Autodesk Fusion 360 part; units mm, degrees
(part 4 of 7)
  spline S47 degree 5 poles (-31.3994, -15.09) (-31.3967, -15.097) (-31.3914, -15.1111) (-31.3834, -15.1322) (-31.3727, -15.1603) (-31.3591, -15.1953) (-31.3454, -15.2302) (-31.3315, -15.265) (-31.3175, -15.2997) (-31.3034, -15.3343) (-31.2892, -15.3688) (-31.2748, -15.4031) (-31.2603, -15.4374) (-31.2457, -15.4715) (-31.2309, -15.5056) (-31.216, -15.5395) (-31.2009, -15.5733) (-31.1857, -15.607) (-31.1704, -15.6406) (-31.155, -15.674) (-31.1394, -15.7073) (-31.1236, -15.7406) (-31.1078, -15.7737) (-31.0917, -15.8066) (-31.0756, -15.8395) (-31.0593, -15.8722) (-31.0429, -15.9048) (-31.0263, -15.9373) (-31.0096, -15.9696) (-30.9927, -16.0018) (-30.9757, -16.0339) (-30.9586, -16.0658) (-30.9413, -16.0976) (-30.9238, -16.1293) (-30.9063, -16.1608) (-30.8885, -16.1922) (-30.8706, -16.2234) (-30.8526, -16.2545) (-30.8344, -16.2855) (-30.8161, -16.3163) (-30.7976, -16.3469) (-30.7789, -16.3774) (-30.7601, -16.4077) (-30.7411, -16.4379) (-30.722, -16.4679) (-30.7027, -16.4977) (-30.6833, -16.5274) (-30.6637, -16.5569) (-30.6439, -16.5863) (-30.6239, -16.6154) (-30.6038, -16.6444) (-30.5835, -16.6732) (-30.563, -16.7018) (-30.5423, -16.7301) (-30.5214, -16.7583) (-30.5003, -16.7862) (-30.4791, -16.814) (-30.4577, -16.8416) (-30.4361, -16.869) (-30.4144, -16.8962) (-30.3923, -16.9231) (-30.37, -16.9497) (-30.3474, -16.9759) (-30.3245, -17.0018) (-30.3014, -17.0274) (-30.2781, -17.0528) (-30.2546, -17.078) (-30.231, -17.103) (-30.2072, -17.1278) (-30.183, -17.1521) (-30.1582, -17.1757) (-30.1377, -17.1938) (-30.1219, -17.2068) (-30.1111, -17.2152) (-30.1057, -17.2194) knots -1 -1 -1 -1 -1 -1 -0.98571429 -0.97142857 -0.95714286 -0.94285714 -0.92857143 -0.91428571 -0.9 -0.88571429 -0.87142857 -0.85714286 -0.84285714 -0.82857143 -0.81428571 -0.8 -0.78571429 -0.77142857 -0.75714286 -0.74285714 -0.72857143 -0.71428571 -0.7 -0.68571429 -0.67142857 -0.65714286 -0.64285714 -0.62857143 -0.61428571 -0.6 -0.58571429 -0.57142857 -0.55714286 -0.54285714 -0.52857143 -0.51428571 -0.5 -0.48571429 -0.47142857 -0.45714286 -0.44285714 -0.42857143 -0.41428571 -0.4 -0.38571429 -0.37142857 -0.35714286 -0.34285714 -0.32857143 -0.31428571 -0.3 -0.28571429 -0.27142857 -0.25714286 -0.24285714 -0.22857143 -0.21428571 -0.2 -0.18571429 -0.17142857 -0.15714286 -0.14285714 -0.12857143 -0.11428571 -0.1 -0.08571429 -0.07142857 -0.05714286 -0.04285714 -0.02857143 -0.01428571 0 0 0 0 0 0
  line L47 (-30.1057, -17.2194) -> (-30.0219, -17.2834)
  arc A95 (-29.9186, -17.9712) -> (-30.0219, -17.2834) centre (-30.3255, -17.6807) ccw
  arc A96 (-29.9186, -17.9712) -> (-30.1974, -18.3752) centre (-17.3506, -26.9445) ccw
  arc A97 (-30.8771, -18.5225) -> (-30.1974, -18.3752) centre (-30.6134, -18.0977) ccw
  line L48 (-30.8771, -18.5225) -> (-30.9667, -18.4669)
  spline S48 degree 5 poles (-30.9667, -18.4669) (-30.9726, -18.4632) (-30.9843, -18.4562) (-31.002, -18.446) (-31.0262, -18.4333) (-31.0571, -18.4184) (-31.0884, -18.4045) (-31.12, -18.391) (-31.1518, -18.3778) (-31.1837, -18.3648) (-31.2157, -18.3519) (-31.2478, -18.3394) (-31.2802, -18.3272) (-31.3127, -18.3153) (-31.3455, -18.3039) (-31.3784, -18.2928) (-31.4115, -18.2821) (-31.4448, -18.2717) (-31.4782, -18.2614) (-31.5117, -18.2514) (-31.5453, -18.2417) (-31.5791, -18.2321) (-31.6129, -18.2228) (-31.6469, -18.2138) (-31.681, -18.205) (-31.7152, -18.1965) (-31.7496, -18.1882) (-31.784, -18.1801) (-31.8186, -18.1722) (-31.8532, -18.1645) (-31.888, -18.1571) (-31.9228, -18.1498) (-31.9577, -18.1428) (-31.9928, -18.1359) (-32.0279, -18.1293) (-32.0631, -18.1229) (-32.0984, -18.1167) (-32.1338, -18.1106) (-32.1692, -18.1048) (-32.2048, -18.0991) (-32.2404, -18.0937) (-32.2761, -18.0884) (-32.3119, -18.0833) (-32.3478, -18.0785) (-32.3837, -18.0737) (-32.4198, -18.0692) (-32.4558, -18.0649) (-32.492, -18.0607) (-32.5282, -18.0567) (-32.5646, -18.0529) (-32.6009, -18.0493) (-32.6374, -18.0459) (-32.6739, -18.0426) (-32.7104, -18.0395) (-32.7471, -18.0365) (-32.7838, -18.0338) (-32.8206, -18.0312) (-32.8574, -18.0288) (-32.8943, -18.0265) (-32.9312, -18.0244) (-32.9682, -18.0225) (-33.0053, -18.0208) (-33.0424, -18.0192) (-33.0796, -18.0178) (-33.1168, -18.0165) (-33.1541, -18.0154) (-33.1914, -18.0145) (-33.2288, -18.0137) (-33.2663, -18.0131) (-33.3038, -18.0127) (-33.3413, -18.0124) (-33.3714, -18.0123) (-33.394, -18.0123) (-33.409, -18.0123) (-33.4166, -18.0123) knots 0 0 0 0 0 0 0.01428571 0.02857143 0.04285714 0.05714286 0.07142857 0.08571429 0.1 0.11428571 0.12857143 0.14285714 0.15714286 0.17142857 0.18571429 0.2 0.21428571 0.22857143 0.24285714 0.25714286 0.27142857 0.28571429 0.3 0.31428571 0.32857143 0.34285714 0.35714286 0.37142857 0.38571429 0.4 0.41428571 0.42857143 0.44285714 0.45714286 0.47142857 0.48571429 0.5 0.51428571 0.52857143 0.54285714 0.55714286 0.57142857 0.58571429 0.6 0.61428571 0.62857143 0.64285714 0.65714286 0.67142857 0.68571429 0.7 0.71428571 0.72857143 0.74285714 0.75714286 0.77142857 0.78571429 0.8 0.81428571 0.82857143 0.84285714 0.85714286 0.87142857 0.88571429 0.9 0.91428571 0.92857143 0.94285714 0.95714286 0.97142857 0.98571429 1 1 1 1 1 1
  arc A98 (-33.4166, -18.0123) -> (-33.8281, -18.7965) centre (-17.3506, -26.9445) ccw
  spline S49 degree 5 poles (-33.8281, -18.7965) (-33.8239, -18.8027) (-33.8153, -18.8152) (-33.8025, -18.8337) (-33.7853, -18.8584) (-33.7638, -18.8892) (-33.7421, -18.9198) (-33.7203, -18.9502) (-33.6985, -18.9806) (-33.6765, -19.0108) (-33.6544, -19.0408) (-33.6322, -19.0708) (-33.6099, -19.1006) (-33.5876, -19.1302) (-33.5651, -19.1597) (-33.5425, -19.1891) (-33.5198, -19.2183) (-33.497, -19.2474) (-33.474, -19.2763) (-33.451, -19.3051) (-33.4279, -19.3337) (-33.4047, -19.3622) (-33.3814, -19.3906) (-33.3579, -19.4187) (-33.3344, -19.4468) (-33.3107, -19.4746) (-33.287, -19.5024) (-33.2631, -19.5299) (-33.2391, -19.5573) (-33.2151, -19.5846) (-33.1909, -19.6116) (-33.1666, -19.6385) (-33.1422, -19.6653) (-33.1177, -19.6918) (-33.0931, -19.7182) (-33.0683, -19.7445) (-33.0435, -19.7705) (-33.0185, -19.7964) (-32.9935, -19.8221) (-32.9683, -19.8476) (-32.943, -19.8729) (-32.9176, -19.8981) (-32.8921, -19.923) (-32.8664, -19.9478) (-32.8407, -19.9723) (-32.8148, -19.9967) (-32.7888, -20.0208) (-32.7627, -20.0448) (-32.7365, -20.0685) (-32.7101, -20.0921) (-32.6837, -20.1154) (-32.657, -20.1385) (-32.6303, -20.1613) (-32.6034, -20.1839) (-32.5764, -20.2062) (-32.5493, -20.2284) (-32.522, -20.2503) (-32.4946, -20.2719) (-32.4671, -20.2934) (-32.4395, -20.3145) (-32.4117, -20.3354) (-32.3836, -20.3558) (-32.3554, -20.3759) (-32.327, -20.3956) (-32.2984, -20.4149) (-32.2697, -20.434) (-32.2408, -20.4528) (-32.2119, -20.4715) (-32.1829, -20.4898) (-32.1536, -20.5076) (-32.1239, -20.5246) (-32.0996, -20.5373) (-32.0812, -20.5461) (-32.0687, -20.5517) (-32.0624, -20.5545) knots -1 -1 -1 -1 -1 -1 -0.98571429 -0.97142857 -0.95714286 -0.94285714 -0.92857143 -0.91428571 -0.9 -0.88571429 -0.87142857 -0.85714286 -0.84285714 -0.82857143 -0.81428571 -0.8 -0.78571429 -0.77142857 -0.75714286 -0.74285714 -0.72857143 -0.71428571 -0.7 -0.68571429 -0.67142857 -0.65714286 -0.64285714 -0.62857143 -0.61428571 -0.6 -0.58571429 -0.57142857 -0.55714286 -0.54285714 -0.52857143 -0.51428571 -0.5 -0.48571429 -0.47142857 -0.45714286 -0.44285714 -0.42857143 -0.41428571 -0.4 -0.38571429 -0.37142857 -0.35714286 -0.34285714 -0.32857143 -0.31428571 -0.3 -0.28571429 -0.27142857 -0.25714286 -0.24285714 -0.22857143 -0.21428571 -0.2 -0.18571429 -0.17142857 -0.15714286 -0.14285714 -0.12857143 -0.11428571 -0.1 -0.08571429 -0.07142857 -0.05714286 -0.04285714 -0.02857143 -0.01428571 0 0 0 0 0 0
  line L49 (-32.0624, -20.5545) -> (-31.9657, -20.5966)
  arc A99 (-31.7009, -21.2397) -> (-31.9657, -20.5966) centre (-32.1655, -21.055) ccw
  arc A100 (-31.7009, -21.2397) -> (-31.8749, -21.6986) centre (-17.3506, -26.9445) ccw
  arc A101 (-32.4996, -22.0043) -> (-31.8749, -21.6986) centre (-32.3452, -21.5288) ccw
  line L50 (-32.4996, -22.0043) -> (-32.5999, -21.9718)
  spline S50 degree 5 poles (-32.5999, -21.9718) (-32.6064, -21.9696) (-32.6195, -21.9656) (-32.6392, -21.9599) (-32.6657, -21.9534) (-32.6992, -21.9464) (-32.733, -21.9403) (-32.7669, -21.9347) (-32.8009, -21.9295) (-32.835, -21.9245) (-32.8691, -21.9198) (-32.9033, -21.9153) (-32.9376, -21.9111) (-32.9721, -21.9074) (-33.0066, -21.9042) (-33.0413, -21.9013) (-33.076, -21.8988) (-33.1108, -21.8966) (-33.1457, -21.8947) (-33.1806, -21.893) (-33.2156, -21.8916) (-33.2506, -21.8904) (-33.2857, -21.8895) (-33.3209, -21.8888) (-33.3561, -21.8884) (-33.3914, -21.8883) (-33.4267, -21.8885) (-33.4621, -21.8889) (-33.4975, -21.8895) (-33.533, -21.8904) (-33.5685, -21.8914) (-33.6041, -21.8927) (-33.6397, -21.8942) (-33.6753, -21.896) (-33.711, -21.898) (-33.7467, -21.9001) (-33.7825, -21.9026) (-33.8183, -21.9052) (-33.8541, -21.908) (-33.89, -21.911) (-33.9259, -21.9142) (-33.9618, -21.9177) (-33.9978, -21.9213) (-34.0338, -21.9251) (-34.0698, -21.9292) (-34.1059, -21.9334) (-34.1419, -21.9378) (-34.1781, -21.9424) (-34.2142, -21.9472) (-34.2504, -21.9522) (-34.2865, -21.9574) (-34.3227, -21.9628) (-34.359, -21.9683) (-34.3952, -21.9741) (-34.4315, -21.98) (-34.4678, -21.9861) (-34.5041, -21.9924) (-34.5404, -21.9989) (-34.5768, -22.0055) (-34.6132, -22.0123) (-34.6496, -22.0193) (-34.686, -22.0265) (-34.7224, -22.0338) (-34.7588, -22.0413) (-34.7953, -22.049) (-34.8317, -22.0569) (-34.8682, -22.0649) (-34.9047, -22.0731) (-34.9412, -22.0815) (-34.9777, -22.09) (-35.0142, -22.0988) (-35.0435, -22.1058) (-35.0654, -22.1112) (-35.08, -22.1149) (-35.0873, -22.1167) knots 0 0 0 0 0 0 0.01428571 0.02857143 0.04285714 0.05714286 0.07142857 0.08571429 0.1 0.11428571 0.12857143 0.14285714 0.15714286 0.17142857 0.18571429 0.2 0.21428571 0.22857143 0.24285714 0.25714286 0.27142857 0.28571429 0.3 0.31428571 0.32857143 0.34285714 0.35714286 0.37142857 0.38571429 0.4 0.41428571 0.42857143 0.44285714 0.45714286 0.47142857 0.48571429 0.5 0.51428571 0.52857143 0.54285714 0.55714286 0.57142857 0.58571429 0.6 0.61428571 0.62857143 0.64285714 0.65714286 0.67142857 0.68571429 0.7 0.71428571 0.72857143 0.74285714 0.75714286 0.77142857 0.78571429 0.8 0.81428571 0.82857143 0.84285714 0.85714286 0.87142857 0.88571429 0.9 0.91428571 0.92857143 0.94285714 0.95714286 0.97142857 0.98571429 1 1 1 1 1 1
  arc A102 (-35.0873, -22.1167) -> (-35.2993, -22.9766) centre (-17.3506, -26.9445) ccw
  spline S51 degree 5 poles (-35.2993, -22.9766) (-35.2936, -22.9816) (-35.2824, -22.9916) (-35.2655, -23.0066) (-35.2429, -23.0265) (-35.2146, -23.0512) (-35.1862, -23.0757) (-35.1578, -23.1001) (-35.1293, -23.1243) (-35.1008, -23.1484) (-35.0721, -23.1723) (-35.0434, -23.196) (-35.0147, -23.2196) (-34.9858, -23.243) (-34.9569, -23.2663) (-34.9279, -23.2894) (-34.8989, -23.3123) (-34.8698, -23.3351) (-34.8406, -23.3577) (-34.8114, -23.3802) (-34.7821, -23.4024) (-34.7527, -23.4245) (-34.7233, -23.4465) (-34.6938, -23.4682) (-34.6642, -23.4898) (-34.6346, -23.5112) (-34.6049, -23.5324) (-34.5751, -23.5535) (-34.5453, -23.5744) (-34.5154, -23.595) (-34.4855, -23.6155) (-34.4554, -23.6358) (-34.4253, -23.656) (-34.3952, -23.6759) (-34.365, -23.6956) (-34.3347, -23.7152) (-34.3043, -23.7345) (-34.2739, -23.7537) (-34.2434, -23.7726) (-34.2129, -23.7914) (-34.1822, -23.8099) (-34.1516, -23.8283) (-34.1208, -23.8464) (-34.09, -23.8643) (-34.0591, -23.8819) (-34.0282, -23.8994) (-33.9971, -23.9166) (-33.9661, -23.9336) (-33.9349, -23.9504) (-33.9037, -23.967) (-33.8724, -23.9833) (-33.8411, -23.9993) (-33.8096, -24.0151) (-33.7781, -24.0306) (-33.7465, -24.0458) (-33.7149, -24.0608) (-33.6832, -24.0755) (-33.6514, -24.09) (-33.6196, -24.1043) (-33.5877, -24.1182) (-33.5557, -24.1318) (-33.5236, -24.1449) (-33.4914, -24.1577) (-33.4591, -24.17) (-33.4267, -24.1819) (-33.3942, -24.1935) (-33.3617, -24.2049) (-33.3292, -24.2161) (-33.2966, -24.227) (-33.2639, -24.2373) (-33.231, -24.2466) (-33.2044, -24.2531) (-33.1843, -24.2573) (-33.1709, -24.2598) (-33.1641, -24.2609) knots -1 -1 -1 -1 -1 -1 -0.98571429 -0.97142857 -0.95714286 -0.94285714 -0.92857143 -0.91428571 -0.9 -0.88571429 -0.87142857 -0.85714286 -0.84285714 -0.82857143 -0.81428571 -0.8 -0.78571429 -0.77142857 -0.75714286 -0.74285714 -0.72857143 -0.71428571 -0.7 -0.68571429 -0.67142857 -0.65714286 -0.64285714 -0.62857143 -0.61428571 -0.6 -0.58571429 -0.57142857 -0.55714286 -0.54285714 -0.52857143 -0.51428571 -0.5 -0.48571429 -0.47142857 -0.45714286 -0.44285714 -0.42857143 -0.41428571 -0.4 -0.38571429 -0.37142857 -0.35714286 -0.34285714 -0.32857143 -0.31428571 -0.3 -0.28571429 -0.27142857 -0.25714286 -0.24285714 -0.22857143 -0.21428571 -0.2 -0.18571429 -0.17142857 -0.15714286 -0.14285714 -0.12857143 -0.11428571 -0.1 -0.08571429 -0.07142857 -0.05714286 -0.04285714 -0.02857143 -0.01428571 0 0 0 0 0 0
  line L51 (-33.1641, -24.2609) -> (-33.0602, -24.2787)
  arc A103 (-32.6491, -24.8397) -> (-33.0602, -24.2787) centre (-33.1444, -24.7715) ccw
  circle A104 centre (-17.3506, -26.9445) radius 2.7
  circle A105 centre (-17.3506, -26.9445) radius 2.7
  circle A106 centre (-17.3506, -26.9445) radius 2.7
  circle A107 centre (-17.3506, -26.9445) radius 4.25
  dimension "d37" = 8.5
  constraint concentric A0 A105
  constraint concentric A105 A106
  constraint concentric A105 A107
  measures "d37" diameter of A107
sketch "Sketch2 (2)" plane through (0, 0, 0) normal (0, 1, 0) x (1, 0, 0)
  circle A0 centre (-38.9137, -5.4395) radius 4.5
  circle A1 centre (-38.9137, -5.4395) radius 6.5
  dimension "d52" = 9
  dimension "d53" = 13
  constraint concentric A0 A1
  measures "d52" diameter of A0
  measures "d53" diameter of A1
extrude "Extrude1'" add sketch "Sketch2 (2)" along normal blind 107 separate body makes body 2
move_body "Move1" bodies 2 to x (0.996195, 0, -0.087156) y (0, 1, 0) z (0.087156, 0, 0.996195) at (25.7661, 0, -8.7245)
move_body "Move2" bodies 2 to x (1, 0, 0) y (0, 1, 0) z (0, 0, 1) at (0, -2, 0)
combine "Combine1" operation add target body 2 tool bodies 1
sketch "Sketch3" plane through (0, 0, 0) normal (1, 0, 0) x (0, 1, 0)
  line L0 (105.0534, -1.0193) -> (-2.1023, -1.0193)
  circle A0 centre (96.2618, -1.0193) radius 1.5
  circle A1 centre (83.5203, -1.0193) radius 1.375
  circle A2 centre (73.2634, -1.0193) radius 1.25
  circle A3 centre (64.1533, -1.0193) radius 1
  circle A4 centre (54.852, -1.0193) radius 1.5
  circle A5 centre (47.2708, -1.0193) radius 1.55
  circle A6 centre (39.3074, -1.0193) radius 1.375
  circle A7 centre (30.7706, -1.0193) radius 1.25
  circle A8 centre (22.0427, -1.0193) radius 1
  circle A9 centre (12.1681, -1.0193) radius 1.5
  circle A10 centre (4.0136, -1.0193) radius 1.5
  dimension "d56" = 3
  dimension "d57" = 2.75
  dimension "d58" = 2.5
  dimension "d59" = 2
  dimension "d60" = 3
  dimension "d61" = 3.1
  dimension "d62" = 2.75
  dimension "d63" = 2.5
  dimension "d64" = 2
  dimension "d65" = 3
  dimension "d66" = 3
  constraint horizontal L0
  constraint coincident L0 A0.centre
  constraint coincident L0 A1.centre
  constraint coincident L0 A2.centre
  constraint coincident L0 A3.centre
  constraint coincident L0 A4.centre
  constraint coincident L0 A5.centre
  constraint coincident L0 A6.centre
  constraint coincident L0 A7.centre
  constraint coincident L0 A8.centre
  constraint coincident L0 A9.centre
  constraint coincident L0 A10.centre
  measures "d56" diameter of A0
  measures "d57" diameter of A1
  measures "d58" diameter of A2
  measures "d59" diameter of A3
  measures "d60" diameter of A4
  measures "d61" diameter of A5
  measures "d62" diameter of A6
  measures "d63" diameter of A7
  measures "d64" diameter of A8
  measures "d65" diameter of A9
  measures "d66" diameter of A10
extrude "Extrude2" cut sketch "Sketch3" against normal blind 17 from surface at -10 bodies 2
component "Rack; Circular Pitch: 4.12283 mm; Num Teeth: 26; Pressure Angle: 20 deg; Backlash: 0.12 mm;" placed x (1, 0, 0) y (0, 1, 0) z (0, 0, 1) at (0, 0, 0)

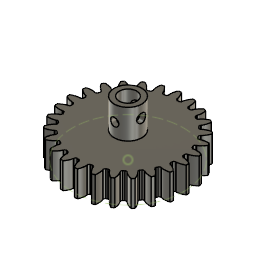
design "Pinion Gear (26t)"
description: Spur Gear; Module: 1.313; Num Teeth: 26; Pressure Angle: 20.0; Backlash: 0.12 mm
Autodesk Fusion 360 part; units mm, degrees
sketch "Sketch1" plane through (0, 0, 0) normal (0, 0, 1) x (1, 0, 0) in component "Spur Gear (26 teeth)"
  circle A0 centre (0, 0) radius 15.4426
  circle A1 centre (0, 0) radius 2.7
extrude "Extrude1" add sketch "Sketch1" along normal blind 8 in component "Spur Gear (26 teeth)"
sketch "Sketch2" plane through (0, 0, 0) normal (0, 0, 1) x (1, 0, 0) in component "Spur Gear (26 teeth)"
  spline S0 degree 5 poles (15.9962, -1.1788) (16.0031, -1.1793) (16.0167, -1.1802) (16.0372, -1.1809) (16.0645, -1.181) (16.0987, -1.1797) (16.1329, -1.1776) (16.1672, -1.1748) (16.2015, -1.1717) (16.2358, -1.1684) (16.27, -1.1649) (16.3044, -1.1611) (16.3387, -1.1569) (16.373, -1.1522) (16.4073, -1.1471) (16.4416, -1.1416) (16.4759, -1.1357) (16.5102, -1.1295) (16.5446, -1.123) (16.5789, -1.1163) (16.6132, -1.1094) (16.6475, -1.1021) (16.6818, -1.0946) (16.7161, -1.0868) (16.7504, -1.0788) (16.7846, -1.0704) (16.8189, -1.0618) (16.8532, -1.053) (16.8874, -1.0439) (16.9217, -1.0346) (16.9559, -1.025) (16.9901, -1.0153) (17.0243, -1.0053) (17.0585, -0.995) (17.0927, -0.9846) (17.1268, -0.9739) (17.161, -0.963) (17.1951, -0.9519) (17.2292, -0.9406) (17.2633, -0.9291) (17.2974, -0.9174) (17.3315, -0.9054) (17.3656, -0.8933) (17.3996, -0.8809) (17.4336, -0.8684) (17.4676, -0.8557) (17.5016, -0.8428) (17.5355, -0.8296) (17.5695, -0.8163) (17.6034, -0.8028) (17.6373, -0.7891) (17.6711, -0.7752) (17.705, -0.7612) (17.7388, -0.7469) (17.7726, -0.7325) (17.8064, -0.7179) (17.8402, -0.7031) (17.8739, -0.6881) (17.9076, -0.673) (17.9413, -0.6577) (17.9749, -0.6422) (18.0086, -0.6265) (18.0422, -0.6106) (18.0758, -0.5946) (18.1093, -0.5784) (18.1428, -0.5621) (18.1763, -0.5455) (18.2098, -0.5288) (18.2432, -0.512) (18.2766, -0.4949) (18.31, -0.4778) (18.3367, -0.4639) (18.3567, -0.4534) (18.37, -0.4463) (18.3767, -0.4428) knots 0 0 0 0 0 0 0.01428571 0.02857143 0.04285714 0.05714286 0.07142857 0.08571429 0.1 0.11428571 0.12857143 0.14285714 0.15714286 0.17142857 0.18571429 0.2 0.21428571 0.22857143 0.24285714 0.25714286 0.27142857 0.28571429 0.3 0.31428571 0.32857143 0.34285714 0.35714286 0.37142857 0.38571429 0.4 0.41428571 0.42857143 0.44285714 0.45714286 0.47142857 0.48571429 0.5 0.51428571 0.52857143 0.54285714 0.55714286 0.57142857 0.58571429 0.6 0.61428571 0.62857143 0.64285714 0.65714286 0.67142857 0.68571429 0.7 0.71428571 0.72857143 0.74285714 0.75714286 0.77142857 0.78571429 0.8 0.81428571 0.82857143 0.84285714 0.85714286 0.87142857 0.88571429 0.9 0.91428571 0.92857143 0.94285714 0.95714286 0.97142857 0.98571429 1 1 1 1 1 1
  spline S1 degree 5 poles (15.9962, 1.1788) (16.0031, 1.1793) (16.0167, 1.1802) (16.0372, 1.1809) (16.0645, 1.181) (16.0987, 1.1797) (16.1329, 1.1776) (16.1672, 1.1748) (16.2015, 1.1717) (16.2358, 1.1684) (16.27, 1.1649) (16.3044, 1.1611) (16.3387, 1.1569) (16.373, 1.1522) (16.4073, 1.1471) (16.4416, 1.1416) (16.4759, 1.1357) (16.5102, 1.1295) (16.5446, 1.123) (16.5789, 1.1163) (16.6132, 1.1094) (16.6475, 1.1021) (16.6818, 1.0946) (16.7161, 1.0868) (16.7504, 1.0788) (16.7846, 1.0704) (16.8189, 1.0618) (16.8532, 1.053) (16.8874, 1.0439) (16.9217, 1.0346) (16.9559, 1.025) (16.9901, 1.0153) (17.0243, 1.0053) (17.0585, 0.995) (17.0927, 0.9846) (17.1268, 0.9739) (17.161, 0.963) (17.1951, 0.9519) (17.2292, 0.9406) (17.2633, 0.9291) (17.2974, 0.9174) (17.3315, 0.9054) (17.3656, 0.8933) (17.3996, 0.8809) (17.4336, 0.8684) (17.4676, 0.8557) (17.5016, 0.8428) (17.5355, 0.8296) (17.5695, 0.8163) (17.6034, 0.8028) (17.6373, 0.7891) (17.6711, 0.7752) (17.705, 0.7612) (17.7388, 0.7469) (17.7726, 0.7325) (17.8064, 0.7179) (17.8402, 0.7031) (17.8739, 0.6881) (17.9076, 0.673) (17.9413, 0.6577) (17.9749, 0.6422) (18.0086, 0.6265) (18.0422, 0.6106) (18.0758, 0.5946) (18.1093, 0.5784) (18.1428, 0.5621) (18.1763, 0.5455) (18.2098, 0.5288) (18.2432, 0.512) (18.2766, 0.4949) (18.31, 0.4778) (18.3367, 0.4639) (18.3567, 0.4534) (18.37, 0.4463) (18.3767, 0.4428) knots 0 0 0 0 0 0 0.01428571 0.02857143 0.04285714 0.05714286 0.07142857 0.08571429 0.1 0.11428571 0.12857143 0.14285714 0.15714286 0.17142857 0.18571429 0.2 0.21428571 0.22857143 0.24285714 0.25714286 0.27142857 0.28571429 0.3 0.31428571 0.32857143 0.34285714 0.35714286 0.37142857 0.38571429 0.4 0.41428571 0.42857143 0.44285714 0.45714286 0.47142857 0.48571429 0.5 0.51428571 0.52857143 0.54285714 0.55714286 0.57142857 0.58571429 0.6 0.61428571 0.62857143 0.64285714 0.65714286 0.67142857 0.68571429 0.7 0.71428571 0.72857143 0.74285714 0.75714286 0.77142857 0.78571429 0.8 0.81428571 0.82857143 0.84285714 0.85714286 0.87142857 0.88571429 0.9 0.91428571 0.92857143 0.94285714 0.95714286 0.97142857 0.98571429 1 1 1 1 1 1
  arc A0 (18.3767, -0.4428) -> (18.3767, 0.4428) centre (0, 0) ccw
  line L0 (15.3909, -1.135) -> (15.9962, -1.1788)
  line L1 (15.3909, 1.135) -> (15.9962, 1.1788)
  line L2 (15.3909, -1.135) -> (15.3909, 1.135)
  point P0 (16.1643, -1.175)
  point P1 (16.3333, -1.1575)
  point P2 (16.5029, -1.1308)
  point P3 (16.6728, -1.0965)
  point P4 (16.8431, -1.0555)
  point P5 (17.0136, -1.0084)
  point P6 (17.1843, -0.9554)
  point P7 (17.355, -0.897)
  point P8 (17.5256, -0.8334)
  point P9 (17.6962, -0.7648)
  point P10 (17.8667, -0.6913)
  point P11 (18.037, -0.6131)
  point P12 (18.207, -0.5302)
  point P13 (16.1643, 1.175)
  point P14 (16.3333, 1.1575)
  point P15 (16.5029, 1.1308)
  point P16 (16.6728, 1.0965)
  point P17 (16.8431, 1.0555)
  point P18 (17.0136, 1.0084)
  point P19 (17.1843, 0.9554)
  point P20 (17.355, 0.897)
  point P21 (17.5256, 0.8334)
  point P22 (17.6962, 0.7648)
  point P23 (17.8667, 0.6913)
  point P24 (18.037, 0.6131)
  point P25 (18.207, 0.5302)
extrude "Extrude2" add sketch "Sketch2" along normal blind 8 in component "Spur Gear (26 teeth)"
fillet "Fillet1" radius 0.5 2 edges at (15.4008, -1.1357, 4) (15.4008, 1.1357, 4) in component "Spur Gear (26 teeth)"
pattern_circular "C-Pattern1" count 26 over 360 about axis through (0, 0, 0) along (0, 0, 1) of "Extrude2", "Fillet1" in component "Spur Gear (26 teeth)"
sketch "Sketch3" plane through (0, 0, 0) normal (0, 0, 1) x (1, 0, 0) in component "Spur Gear (26 teeth)"
  circle A0 centre (0, 0) radius 17.069 construction
sketch "Sketch1 (2)" plane through (0, 0, 8) normal (0, 0, 1) x (-1, 0, 0)
  arc A0 (-32.6491, -24.8397) -> (-32.7083, -25.327) centre (-17.3506, -26.9445) ccw
  arc A1 (-33.2417, -25.7733) -> (-32.7083, -25.327) centre (-33.2055, -25.2746) ccw
  line L0 (-33.2417, -25.7733) -> (-33.3469, -25.7656)
  spline S0 degree 5 poles (-33.3469, -25.7656) (-33.3537, -25.7652) (-33.3673, -25.7643) (-33.3878, -25.7636) (-33.4151, -25.7635) (-33.4493, -25.7648) (-33.4836, -25.7669) (-33.5178, -25.7697) (-33.5521, -25.7728) (-33.5864, -25.7761) (-33.6207, -25.7796) (-33.655, -25.7834) (-33.6893, -25.7876) (-33.7236, -25.7922) (-33.7579, -25.7974) (-33.7922, -25.8029) (-33.8265, -25.8088) (-33.8609, -25.815) (-33.8952, -25.8214) (-33.9295, -25.8282) (-33.9638, -25.8351) (-33.9981, -25.8424) (-34.0324, -25.8499) (-34.0667, -25.8577) (-34.101, -25.8657) (-34.1353, -25.8741) (-34.1695, -25.8827) (-34.2038, -25.8915) (-34.238, -25.9006) (-34.2723, -25.9099) (-34.3065, -25.9194) (-34.3407, -25.9292) (-34.3749, -25.9392) (-34.4091, -25.9494) (-34.4433, -25.9599) (-34.4775, -25.9706) (-34.5116, -25.9815) (-34.5457, -25.9926) (-34.5799, -26.0039) (-34.614, -26.0154) (-34.6481, -26.0271) (-34.6821, -26.0391) (-34.7162, -26.0512) (-34.7502, -26.0635) (-34.7842, -26.0761) (-34.8182, -26.0888) (-34.8522, -26.1017) (-34.8861, -26.1149) (-34.9201, -26.1282) (-34.954, -26.1417) (-34.9879, -26.1554) (-35.0218, -26.1692) (-35.0556, -26.1833) (-35.0894, -26.1976) (-35.1232, -26.212) (-35.157, -26.2266) (-35.1908, -26.2414) (-35.2245, -26.2564) (-35.2582, -26.2715) (-35.2919, -26.2868) (-35.3256, -26.3023) (-35.3592, -26.318) (-35.3928, -26.3339) (-35.4264, -26.3499) (-35.4599, -26.3661) (-35.4934, -26.3824) (-35.5269, -26.399) (-35.5604, -26.4157) (-35.5938, -26.4325) (-35.6272, -26.4495) (-35.6606, -26.4667) (-35.6873, -26.4806) (-35.7073, -26.4911) (-35.7206, -26.4981) (-35.7273, -26.5017) knots 0 0 0 0 0 0 0.01428571 0.02857143 0.04285714 0.05714286 0.07142857 0.08571429 0.1 0.11428571 0.12857143 0.14285714 0.15714286 0.17142857 0.18571429 0.2 0.21428571 0.22857143 0.24285714 0.25714286 0.27142857 0.28571429 0.3 0.31428571 0.32857143 0.34285714 0.35714286 0.37142857 0.38571429 0.4 0.41428571 0.42857143 0.44285714 0.45714286 0.47142857 0.48571429 0.5 0.51428571 0.52857143 0.54285714 0.55714286 0.57142857 0.58571429 0.6 0.61428571 0.62857143 0.64285714 0.65714286 0.67142857 0.68571429 0.7 0.71428571 0.72857143 0.74285714 0.75714286 0.77142857 0.78571429 0.8 0.81428571 0.82857143 0.84285714 0.85714286 0.87142857 0.88571429 0.9 0.91428571 0.92857143 0.94285714 0.95714286 0.97142857 0.98571429 1 1 1 1 1 1
  arc A2 (-35.7273, -26.5017) -> (-35.7273, -27.3873) centre (-17.3506, -26.9445) ccw
  spline S1 degree 5 poles (-35.7273, -27.3873) (-35.7206, -27.3908) (-35.7073, -27.3979) (-35.6873, -27.4084) (-35.6606, -27.4222) (-35.6272, -27.4394) (-35.5938, -27.4565) (-35.5604, -27.4733) (-35.5269, -27.49) (-35.4934, -27.5066) (-35.4599, -27.5229) (-35.4264, -27.5391) (-35.3928, -27.5551) (-35.3592, -27.571) (-35.3256, -27.5866) (-35.2919, -27.6021) (-35.2582, -27.6175) (-35.2245, -27.6326) (-35.1908, -27.6476) (-35.157, -27.6624) (-35.1232, -27.677) (-35.0894, -27.6914) (-35.0556, -27.7057) (-35.0218, -27.7197) (-34.9879, -27.7336) (-34.954, -27.7473) (-34.9201, -27.7608) (-34.8861, -27.7741) (-34.8522, -27.7872) (-34.8182, -27.8002) (-34.7842, -27.8129) (-34.7502, -27.8254) (-34.7162, -27.8378) (-34.6821, -27.8499) (-34.6481, -27.8618) (-34.614, -27.8736) (-34.5799, -27.8851) (-34.5457, -27.8964) (-34.5116, -27.9075) (-34.4775, -27.9184) (-34.4433, -27.9291) (-34.4091, -27.9395) (-34.3749, -27.9498) (-34.3407, -27.9598) (-34.3065, -27.9695) (-34.2723, -27.9791) (-34.238, -27.9884) (-34.2038, -27.9975) (-34.1695, -28.0063) (-34.1353, -28.0149) (-34.101, -28.0233) (-34.0667, -28.0313) (-34.0324, -28.0391) (-33.9981, -28.0466) (-33.9638, -28.0538) (-33.9295, -28.0608) (-33.8952, -28.0675) (-33.8609, -28.074) (-33.8265, -28.0802) (-33.7922, -28.0861) (-33.7579, -28.0916) (-33.7236, -28.0967) (-33.6893, -28.1014) (-33.655, -28.1056) (-33.6207, -28.1094) (-33.5864, -28.1129) (-33.5521, -28.1162) (-33.5178, -28.1193) (-33.4836, -28.1221) (-33.4493, -28.1242) (-33.4151, -28.1254) (-33.3878, -28.1254) (-33.3673, -28.1247) (-33.3537, -28.1238) (-33.3469, -28.1233) knots -1 -1 -1 -1 -1 -1 -0.98571429 -0.97142857 -0.95714286 -0.94285714 -0.92857143 -0.91428571 -0.9 -0.88571429 -0.87142857 -0.85714286 -0.84285714 -0.82857143 -0.81428571 -0.8 -0.78571429 -0.77142857 -0.75714286 -0.74285714 -0.72857143 -0.71428571 -0.7 -0.68571429 -0.67142857 -0.65714286 -0.64285714 -0.62857143 -0.61428571 -0.6 -0.58571429 -0.57142857 -0.55714286 -0.54285714 -0.52857143 -0.51428571 -0.5 -0.48571429 -0.47142857 -0.45714286 -0.44285714 -0.42857143 -0.41428571 -0.4 -0.38571429 -0.37142857 -0.35714286 -0.34285714 -0.32857143 -0.31428571 -0.3 -0.28571429 -0.27142857 -0.25714286 -0.24285714 -0.22857143 -0.21428571 -0.2 -0.18571429 -0.17142857 -0.15714286 -0.14285714 -0.12857143 -0.11428571 -0.1 -0.08571429 -0.07142857 -0.05714286 -0.04285714 -0.02857143 -0.01428571 0 0 0 0 0 0
  line L1 (-33.3469, -28.1233) -> (-33.2417, -28.1157)
  arc A3 (-32.7083, -28.562) -> (-33.2417, -28.1157) centre (-33.2055, -28.6144) ccw
  arc A4 (-32.7083, -28.562) -> (-32.6491, -29.0493) centre (-17.3506, -26.9445) ccw
  arc A5 (-33.0602, -29.6103) -> (-32.6491, -29.0493) centre (-33.1444, -29.1174) ccw
  line L2 (-33.0602, -29.6103) -> (-33.1641, -29.6281)
  spline S2 degree 5 poles (-33.1641, -29.6281) (-33.1709, -29.6292) (-33.1843, -29.6317) (-33.2044, -29.6358) (-33.231, -29.6423) (-33.2639, -29.6517) (-33.2966, -29.662) (-33.3292, -29.6729) (-33.3617, -29.6841) (-33.3942, -29.6955) (-33.4267, -29.7071) (-33.4591, -29.719) (-33.4914, -29.7313) (-33.5236, -29.744) (-33.5557, -29.7572) (-33.5877, -29.7708) (-33.6196, -29.7847) (-33.6514, -29.799) (-33.6832, -29.8135) (-33.7149, -29.8282) (-33.7465, -29.8432) (-33.7781, -29.8584) (-33.8096, -29.8739) (-33.8411, -29.8897) (-33.8724, -29.9057) (-33.9037, -29.922) (-33.9349, -29.9386) (-33.9661, -29.9553) (-33.9971, -29.9724) (-34.0282, -29.9896) (-34.0591, -30.007) (-34.09, -30.0247) (-34.1208, -30.0426) (-34.1516, -30.0607) (-34.1822, -30.0791) (-34.2129, -30.0976) (-34.2434, -30.1163) (-34.2739, -30.1353) (-34.3043, -30.1544) (-34.3347, -30.1738) (-34.365, -30.1933) (-34.3952, -30.2131) (-34.4253, -30.233) (-34.4554, -30.2531) (-34.4855, -30.2734) (-34.5154, -30.2939) (-34.5453, -30.3146) (-34.5751, -30.3355) (-34.6049, -30.3565) (-34.6346, -30.3778) (-34.6642, -30.3992) (-34.6938, -30.4208) (-34.7233, -30.4425) (-34.7527, -30.4644) (-34.7821, -30.4865) (-34.8114, -30.5088) (-34.8406, -30.5313) (-34.8698, -30.5539) (-34.8989, -30.5766) (-34.9279, -30.5996) (-34.9569, -30.6227) (-34.9858, -30.6459) (-35.0147, -30.6694) (-35.0434, -30.693) (-35.0721, -30.7167) (-35.1008, -30.7406) (-35.1293, -30.7647) (-35.1578, -30.7889) (-35.1862, -30.8133) (-35.2146, -30.8378) (-35.2429, -30.8625) (-35.2655, -30.8824) (-35.2824, -30.8973) (-35.2936, -30.9073) (-35.2993, -30.9124) knots 0 0 0 0 0 0 0.01428571 0.02857143 0.04285714 0.05714286 0.07142857 0.08571429 0.1 0.11428571 0.12857143 0.14285714 0.15714286 0.17142857 0.18571429 0.2 0.21428571 0.22857143 0.24285714 0.25714286 0.27142857 0.28571429 0.3 0.31428571 0.32857143 0.34285714 0.35714286 0.37142857 0.38571429 0.4 0.41428571 0.42857143 0.44285714 0.45714286 0.47142857 0.48571429 0.5 0.51428571 0.52857143 0.54285714 0.55714286 0.57142857 0.58571429 0.6 0.61428571 0.62857143 0.64285714 0.65714286 0.67142857 0.68571429 0.7 0.71428571 0.72857143 0.74285714 0.75714286 0.77142857 0.78571429 0.8 0.81428571 0.82857143 0.84285714 0.85714286 0.87142857 0.88571429 0.9 0.91428571 0.92857143 0.94285714 0.95714286 0.97142857 0.98571429 1 1 1 1 1 1
  arc A6 (-35.2993, -30.9124) -> (-35.0873, -31.7723) centre (-17.3506, -26.9445) ccw
  spline S3 degree 5 poles (-35.0873, -31.7723) (-35.08, -31.7741) (-35.0654, -31.7777) (-35.0435, -31.7831) (-35.0142, -31.7902) (-34.9777, -31.7989) (-34.9412, -31.8075) (-34.9047, -31.8158) (-34.8682, -31.824) (-34.8317, -31.8321) (-34.7953, -31.8399) (-34.7588, -31.8476) (-34.7224, -31.8552) (-34.686, -31.8625) (-34.6496, -31.8697) (-34.6132, -31.8767) (-34.5768, -31.8835) (-34.5404, -31.8901) (-34.5041, -31.8966) (-34.4678, -31.9029) (-34.4315, -31.909) (-34.3952, -31.9149) (-34.359, -31.9206) (-34.3227, -31.9262) (-34.2865, -31.9316) (-34.2504, -31.9367) (-34.2142, -31.9417) (-34.1781, -31.9465) (-34.1419, -31.9512) (-34.1059, -31.9556) (-34.0698, -31.9598) (-34.0338, -31.9638) (-33.9978, -31.9677) (-33.9618, -31.9713) (-33.9259, -31.9747) (-33.89, -31.978) (-33.8541, -31.981) (-33.8183, -31.9838) (-33.7825, -31.9864) (-33.7467, -31.9888) (-33.711, -31.991) (-33.6753, -31.993) (-33.6397, -31.9947) (-33.6041, -31.9963) (-33.5685, -31.9976) (-33.533, -31.9986) (-33.4975, -31.9995) (-33.4621, -32.0001) (-33.4267, -32.0005) (-33.3914, -32.0006) (-33.3561, -32.0005) (-33.3209, -32.0002) (-33.2857, -31.9995) (-33.2506, -31.9986) (-33.2156, -31.9974) (-33.1806, -31.996) (-33.1457, -31.9943) (-33.1108, -31.9923) (-33.076, -31.9902) (-33.0413, -31.9877) (-33.0066, -31.9848) (-32.9721, -31.9816) (-32.9376, -31.9779) (-32.9033, -31.9737) (-32.8691, -31.9692) (-32.835, -31.9644) (-32.8009, -31.9594) (-32.7669, -31.9542) (-32.733, -31.9487) (-32.6992, -31.9426) (-32.6657, -31.9356) (-32.6392, -31.929) (-32.6195, -31.9234) (-32.6064, -31.9193) (-32.5999, -31.9172) knots -1 -1 -1 -1 -1 -1 -0.98571429 -0.97142857 -0.95714286 -0.94285714 -0.92857143 -0.91428571 -0.9 -0.88571429 -0.87142857 -0.85714286 -0.84285714 -0.82857143 -0.81428571 -0.8 -0.78571429 -0.77142857 -0.75714286 -0.74285714 -0.72857143 -0.71428571 -0.7 -0.68571429 -0.67142857 -0.65714286 -0.64285714 -0.62857143 -0.61428571 -0.6 -0.58571429 -0.57142857 -0.55714286 -0.54285714 -0.52857143 -0.51428571 -0.5 -0.48571429 -0.47142857 -0.45714286 -0.44285714 -0.42857143 -0.41428571 -0.4 -0.38571429 -0.37142857 -0.35714286 -0.34285714 -0.32857143 -0.31428571 -0.3 -0.28571429 -0.27142857 -0.25714286 -0.24285714 -0.22857143 -0.21428571 -0.2 -0.18571429 -0.17142857 -0.15714286 -0.14285714 -0.12857143 -0.11428571 -0.1 -0.08571429 -0.07142857 -0.05714286 -0.04285714 -0.02857143 -0.01428571 0 0 0 0 0 0
  line L3 (-32.5999, -31.9172) -> (-32.4996, -31.8847)
  arc A7 (-31.8749, -32.1904) -> (-32.4996, -31.8847) centre (-32.3452, -32.3602) ccw
  arc A8 (-31.8749, -32.1904) -> (-31.7009, -32.6493) centre (-17.3506, -26.9445) ccw
  arc A9 (-31.9657, -33.2924) -> (-31.7009, -32.6493) centre (-32.1655, -32.834) ccw
  line L4 (-31.9657, -33.2924) -> (-32.0624, -33.3345)
  spline S4 degree 5 poles (-32.0624, -33.3345) (-32.0687, -33.3372) (-32.0812, -33.3428) (-32.0996, -33.3517) (-32.1239, -33.3644) (-32.1536, -33.3813) (-32.1829, -33.3992) (-32.2119, -33.4175) (-32.2408, -33.4362) (-32.2697, -33.455) (-32.2984, -33.4741) (-32.327, -33.4934) (-32.3554, -33.5131) (-32.3836, -33.5331) (-32.4117, -33.5536) (-32.4395, -33.5744) (-32.4671, -33.5956) (-32.4946, -33.617) (-32.522, -33.6387) (-32.5493, -33.6606) (-32.5764, -33.6827) (-32.6034, -33.7051) (-32.6303, -33.7277) (-32.657, -33.7505) (-32.6837, -33.7736) (-32.7101, -33.7969) (-32.7365, -33.8204) (-32.7627, -33.8442) (-32.7888, -33.8681) (-32.8148, -33.8923) (-32.8407, -33.9167) (-32.8664, -33.9412) (-32.8921, -33.966) (-32.9176, -33.9909) (-32.943, -34.016) (-32.9683, -34.0414) (-32.9935, -34.0669) (-33.0185, -34.0926) (-33.0435, -34.1185) (-33.0683, -34.1445) (-33.0931, -34.1707) (-33.1177, -34.1971) (-33.1422, -34.2237) (-33.1666, -34.2504) (-33.1909, -34.2773) (-33.2151, -34.3044) (-33.2391, -34.3317) (-33.2631, -34.3591) (-33.287, -34.3866) (-33.3107, -34.4143) (-33.3344, -34.4422) (-33.3579, -34.4702) (-33.3814, -34.4984) (-33.4047, -34.5268) (-33.4279, -34.5552) (-33.451, -34.5839) (-33.474, -34.6127) (-33.497, -34.6416) (-33.5198, -34.6707) (-33.5425, -34.6999) (-33.5651, -34.7293) (-33.5876, -34.7588) (-33.6099, -34.7884) (-33.6322, -34.8182) (-33.6544, -34.8481) (-33.6765, -34.8782) (-33.6985, -34.9084) (-33.7203, -34.9387) (-33.7421, -34.9692) (-33.7638, -34.9998) (-33.7853, -35.0305) (-33.8025, -35.0552) (-33.8153, -35.0738) (-33.8239, -35.0862) (-33.8281, -35.0924) knots 0 0 0 0 0 0 0.01428571 0.02857143 0.04285714 0.05714286 0.07142857 0.08571429 0.1 0.11428571 0.12857143 0.14285714 0.15714286 0.17142857 0.18571429 0.2 0.21428571 0.22857143 0.24285714 0.25714286 0.27142857 0.28571429 0.3 0.31428571 0.32857143 0.34285714 0.35714286 0.37142857 0.38571429 0.4 0.41428571 0.42857143 0.44285714 0.45714286 0.47142857 0.48571429 0.5 0.51428571 0.52857143 0.54285714 0.55714286 0.57142857 0.58571429 0.6 0.61428571 0.62857143 0.64285714 0.65714286 0.67142857 0.68571429 0.7 0.71428571 0.72857143 0.74285714 0.75714286 0.77142857 0.78571429 0.8 0.81428571 0.82857143 0.84285714 0.85714286 0.87142857 0.88571429 0.9 0.91428571 0.92857143 0.94285714 0.95714286 0.97142857 0.98571429 1 1 1 1 1 1
  arc A10 (-33.8281, -35.0924) -> (-33.4166, -35.8767) centre (-17.3506, -26.9445) ccw
  spline S5 degree 5 poles (-33.4166, -35.8767) (-33.409, -35.8767) (-33.394, -35.8767) (-33.3714, -35.8767) (-33.3413, -35.8766) (-33.3038, -35.8763) (-33.2663, -35.8759) (-33.2288, -35.8753) (-33.1914, -35.8745) (-33.1541, -35.8736) (-33.1168, -35.8725) (-33.0796, -35.8712) (-33.0424, -35.8698) (-33.0053, -35.8682) (-32.9682, -35.8665) (-32.9312, -35.8645) (-32.8943, -35.8625) (-32.8574, -35.8602) (-32.8206, -35.8578) (-32.7838, -35.8552) (-32.7471, -35.8524) (-32.7104, -35.8495) (-32.6739, -35.8464) (-32.6374, -35.8431) (-32.6009, -35.8397) (-32.5646, -35.836) (-32.5282, -35.8322) (-32.492, -35.8283) (-32.4558, -35.8241) (-32.4198, -35.8198) (-32.3837, -35.8152) (-32.3478, -35.8105) (-32.3119, -35.8056) (-32.2761, -35.8006) (-32.2404, -35.7953) (-32.2048, -35.7898) (-32.1692, -35.7842) (-32.1338, -35.7783) (-32.0984, -35.7723) (-32.0631, -35.7661) (-32.0279, -35.7597) (-31.9928, -35.753) (-31.9577, -35.7462) (-31.9228, -35.7392) (-31.888, -35.7319) (-31.8532, -35.7245) (-31.8186, -35.7168) (-31.784, -35.7089) (-31.7496, -35.7008) (-31.7152, -35.6925) (-31.681, -35.684) (-31.6469, -35.6752) (-31.6129, -35.6661) (-31.5791, -35.6568) (-31.5453, -35.6473) (-31.5117, -35.6375) (-31.4782, -35.6275) (-31.4448, -35.6173) (-31.4115, -35.6069) (-31.3784, -35.5961) (-31.3455, -35.5851) (-31.3127, -35.5736) (-31.2802, -35.5618) (-31.2478, -35.5496) (-31.2157, -35.537) (-31.1837, -35.5242) (-31.1518, -35.5112) (-31.12, -35.498) (-31.0884, -35.4845) (-31.0571, -35.4705) (-31.0262, -35.4557) (-31.002, -35.443) (-30.9843, -35.4328) (-30.9726, -35.4257) (-30.9667, -35.4221) knots -1 -1 -1 -1 -1 -1 -0.98571429 -0.97142857 -0.95714286 -0.94285714 -0.92857143 -0.91428571 -0.9 -0.88571429 -0.87142857 -0.85714286 -0.84285714 -0.82857143 -0.81428571 -0.8 -0.78571429 -0.77142857 -0.75714286 -0.74285714 -0.72857143 -0.71428571 -0.7 -0.68571429 -0.67142857 -0.65714286 -0.64285714 -0.62857143 -0.61428571 -0.6 -0.58571429 -0.57142857 -0.55714286 -0.54285714 -0.52857143 -0.51428571 -0.5 -0.48571429 -0.47142857 -0.45714286 -0.44285714 -0.42857143 -0.41428571 -0.4 -0.38571429 -0.37142857 -0.35714286 -0.34285714 -0.32857143 -0.31428571 -0.3 -0.28571429 -0.27142857 -0.25714286 -0.24285714 -0.22857143 -0.21428571 -0.2 -0.18571429 -0.17142857 -0.15714286 -0.14285714 -0.12857143 -0.11428571 -0.1 -0.08571429 -0.07142857 -0.05714286 -0.04285714 -0.02857143 -0.01428571 0 0 0 0 0 0
  line L5 (-30.9667, -35.4221) -> (-30.8771, -35.3665)
  arc A11 (-30.1974, -35.5138) -> (-30.8771, -35.3665) centre (-30.6134, -35.7913) ccw
  arc A12 (-30.1974, -35.5138) -> (-29.9186, -35.9178) centre (-17.3506, -26.9445) ccw
  arc A13 (-30.0219, -36.6055) -> (-29.9186, -35.9178) centre (-30.3255, -36.2083) ccw
  line L6 (-30.0219, -36.6055) -> (-30.1057, -36.6696)
  spline S6 degree 5 poles (-30.1057, -36.6696) (-30.1111, -36.6737) (-30.1219, -36.6822) (-30.1377, -36.6952) (-30.1582, -36.7133) (-30.183, -36.7369) (-30.2072, -36.7612) (-30.231, -36.786) (-30.2546, -36.811) (-30.2781, -36.8362) (-30.3014, -36.8616) (-30.3245, -36.8872) (-30.3474, -36.9131) (-30.37, -36.9393) (-30.3923, -36.9659) (-30.4144, -36.9928) (-30.4361, -37.02) (-30.4577, -37.0474) (-30.4791, -37.075) (-30.5003, -37.1027) (-30.5214, -37.1307) (-30.5423, -37.1589) (-30.563, -37.1872) (-30.5835, -37.2158) (-30.6038, -37.2446) (-30.6239, -37.2735) (-30.6439, -37.3027) (-30.6637, -37.332) (-30.6833, -37.3616) (-30.7027, -37.3912) (-30.722, -37.4211) (-30.7411, -37.4511) (-30.7601, -37.4812) (-30.7789, -37.5116) (-30.7976, -37.5421) (-30.8161, -37.5727) (-30.8344, -37.6035) (-30.8526, -37.6344) (-30.8706, -37.6655) (-30.8885, -37.6968) (-30.9063, -37.7282) (-30.9238, -37.7597) (-30.9413, -37.7913) (-30.9586, -37.8232) (-30.9757, -37.8551) (-30.9927, -37.8872) (-31.0096, -37.9194) (-31.0263, -37.9517) (-31.0429, -37.9842) (-31.0593, -38.0168) (-31.0756, -38.0495) (-31.0917, -38.0823) (-31.1078, -38.1153) (-31.1236, -38.1484) (-31.1394, -38.1816) (-31.155, -38.215) (-31.1704, -38.2484) (-31.1857, -38.282) (-31.2009, -38.3157) (-31.216, -38.3495) (-31.2309, -38.3834) (-31.2457, -38.4175) (-31.2603, -38.4516) (-31.2748, -38.4859) (-31.2892, -38.5202) (-31.3034, -38.5547) (-31.3175, -38.5893) (-31.3315, -38.624) (-31.3454, -38.6588) (-31.3591, -38.6937) (-31.3727, -38.7287) (-31.3834, -38.7568) (-31.3914, -38.7779) (-31.3967, -38.792) (-31.3994, -38.799) knots 0 0 0 0 0 0 0.01428571 0.02857143 0.04285714 0.05714286 0.07142857 0.08571429 0.1 0.11428571 0.12857143 0.14285714 0.15714286 0.17142857 0.18571429 0.2 0.21428571 0.22857143 0.24285714 0.25714286 0.27142857 0.28571429 0.3 0.31428571 0.32857143 0.34285714 0.35714286 0.37142857 0.38571429 0.4 0.41428571 0.42857143 0.44285714 0.45714286 0.47142857 0.48571429 0.5 0.51428571 0.52857143 0.54285714 0.55714286 0.57142857 0.58571429 0.6 0.61428571 0.62857143 0.64285714 0.65714286 0.67142857 0.68571429 0.7 0.71428571 0.72857143 0.74285714 0.75714286 0.77142857 0.78571429 0.8 0.81428571 0.82857143 0.84285714 0.85714286 0.87142857 0.88571429 0.9 0.91428571 0.92857143 0.94285714 0.95714286 0.97142857 0.98571429 1 1 1 1 1 1
  arc A14 (-31.3994, -38.799) -> (-30.8121, -39.4619) centre (-17.3506, -26.9445) ccw
  spline S7 degree 5 poles (-30.8121, -39.4619) (-30.8048, -39.4602) (-30.7901, -39.4566) (-30.7682, -39.4512) (-30.739, -39.4439) (-30.7027, -39.4346) (-30.6664, -39.4252) (-30.6302, -39.4156) (-30.594, -39.406) (-30.558, -39.3961) (-30.5221, -39.3861) (-30.4862, -39.376) (-30.4505, -39.3657) (-30.4148, -39.3553) (-30.3792, -39.3447) (-30.3438, -39.334) (-30.3084, -39.3232) (-30.2731, -39.3121) (-30.2379, -39.301) (-30.2029, -39.2897) (-30.1679, -39.2782) (-30.133, -39.2666) (-30.0982, -39.2548) (-30.0636, -39.2429) (-30.029, -39.2308) (-29.9946, -39.2186) (-29.9602, -39.2062) (-29.926, -39.1937) (-29.8919, -39.181) (-29.8579, -39.1681) (-29.824, -39.1551) (-29.7902, -39.142) (-29.7566, -39.1286) (-29.723, -39.1151) (-29.6896, -39.1015) (-29.6563, -39.0876) (-29.6232, -39.0736) (-29.5901, -39.0595) (-29.5572, -39.0452) (-29.5244, -39.0307) (-29.4918, -39.016) (-29.4593, -39.0012) (-29.4269, -38.9862) (-29.3946, -38.971) (-29.3626, -38.9556) (-29.3306, -38.94) (-29.2988, -38.9243) (-29.2671, -38.9084) (-29.2356, -38.8923) (-29.2043, -38.876) (-29.1731, -38.8595) (-29.1421, -38.8428) (-29.1112, -38.8259) (-29.0806, -38.8088) (-29.0501, -38.7914) (-29.0198, -38.7739) (-28.9897, -38.7562) (-28.9597, -38.7383) (-28.9299, -38.7201) (-28.9003, -38.7018) (-28.871, -38.6832) (-28.8419, -38.6642) (-28.8131, -38.645) (-28.7847, -38.6254) (-28.7564, -38.6055) (-28.7284, -38.5854) (-28.7006, -38.5651) (-28.6729, -38.5447) (-28.6454, -38.524) (-28.6184, -38.503) (-28.592, -38.4812) (-28.5715, -38.463) (-28.5567, -38.4489) (-28.547, -38.4392) (-28.5423, -38.4343) knots -1 -1 -1 -1 -1 -1 -0.98571429 -0.97142857 -0.95714286 -0.94285714 -0.92857143 -0.91428571 -0.9 -0.88571429 -0.87142857 -0.85714286 -0.84285714 -0.82857143 -0.81428571 -0.8 -0.78571429 -0.77142857 -0.75714286 -0.74285714 -0.72857143 -0.71428571 -0.7 -0.68571429 -0.67142857 -0.65714286 -0.64285714 -0.62857143 -0.61428571 -0.6 -0.58571429 -0.57142857 -0.55714286 -0.54285714 -0.52857143 -0.51428571 -0.5 -0.48571429 -0.47142857 -0.45714286 -0.44285714 -0.42857143 -0.41428571 -0.4 -0.38571429 -0.37142857 -0.35714286 -0.34285714 -0.32857143 -0.31428571 -0.3 -0.28571429 -0.27142857 -0.25714286 -0.24285714 -0.22857143 -0.21428571 -0.2 -0.18571429 -0.17142857 -0.15714286 -0.14285714 -0.12857143 -0.11428571 -0.1 -0.08571429 -0.07142857 -0.05714286 -0.04285714 -0.02857143 -0.01428571 0 0 0 0 0 0
  line L7 (-28.5423, -38.4343) -> (-28.4686, -38.3589)
  arc A15 (-27.7734, -38.3392) -> (-28.4686, -38.3589) centre (-28.1108, -38.7082) ccw
  arc A16 (-27.7734, -38.3392) -> (-27.406, -38.6647) centre (-17.3506, -26.9445) ccw
  arc A17 (-27.3417, -39.3572) -> (-27.406, -38.6647) centre (-27.7315, -39.0442) ccw
  line L8 (-27.3417, -39.3572) -> (-27.4077, -39.4395)
  spline S8 degree 5 poles (-27.4077, -39.4395) (-27.412, -39.4448) (-27.4204, -39.4556) (-27.4326, -39.472) (-27.4482, -39.4945) (-27.4666, -39.5233) (-27.4843, -39.5527) (-27.5015, -39.5825) (-27.5184, -39.6124) (-27.5352, -39.6425) (-27.5518, -39.6727) (-27.5681, -39.7031) (-27.5841, -39.7338) (-27.5998, -39.7646) (-27.6151, -39.7958) (-27.63, -39.8272) (-27.6447, -39.8588) (-27.6591, -39.8905) (-27.6732, -39.9224) (-27.6872, -39.9545) (-27.701, -39.9867) (-27.7145, -40.019) (-27.7278, -40.0515) (-27.7409, -40.0842) (-27.7537, -40.117) (-27.7663, -40.1499) (-27.7787, -40.183) (-27.7909, -40.2162) (-27.8029, -40.2496) (-27.8147, -40.283) (-27.8263, -40.3166) (-27.8377, -40.3503) (-27.8489, -40.3842) (-27.8599, -40.4181) (-27.8707, -40.4522) (-27.8813, -40.4864) (-27.8917, -40.5206) (-27.902, -40.555) (-27.9121, -40.5896) (-27.9219, -40.6242) (-27.9317, -40.6589) (-27.9412, -40.6937) (-27.9505, -40.7286) (-27.9597, -40.7636) (-27.9687, -40.7987) (-27.9776, -40.834) (-27.9862, -40.8693) (-27.9947, -40.9047) (-28.003, -40.9402) (-28.0112, -40.9757) (-28.0192, -41.0114) (-28.027, -41.0472) (-28.0346, -41.083) (-28.0421, -41.1189) (-28.0495, -41.155) (-28.0566, -41.1911) (-28.0636, -41.2272) (-28.0705, -41.2635) (-28.0771, -41.2999) (-28.0837, -41.3363) (-28.09, -41.3728) (-28.0962, -41.4094) (-28.1023, -41.446) (-28.1082, -41.4828) (-28.1139, -41.5196) (-28.1195, -41.5565) (-28.1249, -41.5934) (-28.1302, -41.6304) (-28.1353, -41.6675) (-28.1403, -41.7047) (-28.1451, -41.7419) (-28.1488, -41.7718) (-28.1515, -41.7942) (-28.1533, -41.8092) (-28.1542, -41.8166) knots 0 0 0 0 0 0 0.01428571 0.02857143 0.04285714 0.05714286 0.07142857 0.08571429 0.1 0.11428571 0.12857143 0.14285714 0.15714286 0.17142857 0.18571429 0.2 0.21428571 0.22857143 0.24285714 0.25714286 0.27142857 0.28571429 0.3 0.31428571 0.32857143 0.34285714 0.35714286 0.37142857 0.38571429 0.4 0.41428571 0.42857143 0.44285714 0.45714286 0.47142857 0.48571429 0.5 0.51428571 0.52857143 0.54285714 0.55714286 0.57142857 0.58571429 0.6 0.61428571 0.62857143 0.64285714 0.65714286 0.67142857 0.68571429 0.7 0.71428571 0.72857143 0.74285714 0.75714286 0.77142857 0.78571429 0.8 0.81428571 0.82857143 0.84285714 0.85714286 0.87142857 0.88571429 0.9 0.91428571 0.92857143 0.94285714 0.95714286 0.97142857 0.98571429 1 1 1 1 1 1
  arc A18 (-28.1542, -41.8166) -> (-27.4253, -42.3197) centre (-17.3506, -26.9445) ccw
  spline S9 degree 5 poles (-27.4253, -42.3197) (-27.4186, -42.3163) (-27.4053, -42.3093) (-27.3853, -42.2988) (-27.3587, -42.2847) (-27.3256, -42.267) (-27.2926, -42.2492) (-27.2597, -42.2313) (-27.227, -42.2132) (-27.1943, -42.195) (-27.1618, -42.1767) (-27.1295, -42.1583) (-27.0972, -42.1398) (-27.0651, -42.1211) (-27.0331, -42.1024) (-27.0012, -42.0835) (-26.9694, -42.0645) (-26.9378, -42.0453) (-26.9063, -42.0261) (-26.875, -42.0067) (-26.8438, -41.9872) (-26.8127, -41.9676) (-26.7818, -41.9478) (-26.751, -41.9279) (-26.7203, -41.908) (-26.6898, -41.8878) (-26.6594, -41.8676) (-26.6292, -41.8472) (-26.5991, -41.8267) (-26.5691, -41.8061) (-26.5393, -41.7854) (-26.5097, -41.7645) (-26.4802, -41.7435) (-26.4509, -41.7224) (-26.4217, -41.7011) (-26.3927, -41.6797) (-26.3638, -41.6582) (-26.3351, -41.6366) (-26.3066, -41.6148) (-26.2783, -41.5929) (-26.2501, -41.5708) (-26.222, -41.5486) (-26.1942, -41.5263) (-26.1665, -41.5038) (-26.1391, -41.4812) (-26.1118, -41.4585) (-26.0847, -41.4356) (-26.0577, -41.4125) (-26.031, -41.3894) (-26.0044, -41.366) (-25.9781, -41.3426) (-25.952, -41.3189) (-25.9261, -41.2951) (-25.9004, -41.2712) (-25.875, -41.2471) (-25.8498, -41.2228) (-25.8248, -41.1984) (-25.7999, -41.1738) (-25.7753, -41.1491) (-25.751, -41.1242) (-25.7269, -41.0991) (-25.7033, -41.0737) (-25.6799, -41.0481) (-25.657, -41.0223) (-25.6344, -40.9962) (-25.612, -40.97) (-25.5898, -40.9437) (-25.5678, -40.9172) (-25.5461, -40.8906) (-25.5248, -40.8636) (-25.5044, -40.8362) (-25.4889, -40.8137) (-25.4779, -40.7964) (-25.4708, -40.7847) (-25.4673, -40.7788) knots -1 -1 -1 -1 -1 -1 -0.98571429 -0.97142857 -0.95714286 -0.94285714 -0.92857143 -0.91428571 -0.9 -0.88571429 -0.87142857 -0.85714286 -0.84285714 -0.82857143 -0.81428571 -0.8 -0.78571429 -0.77142857 -0.75714286 -0.74285714 -0.72857143 -0.71428571 -0.7 -0.68571429 -0.67142857 -0.65714286 -0.64285714 -0.62857143 -0.61428571 -0.6 -0.58571429 -0.57142857 -0.55714286 -0.54285714 -0.52857143 -0.51428571 -0.5 -0.48571429 -0.47142857 -0.45714286 -0.44285714 -0.42857143 -0.41428571 -0.4 -0.38571429 -0.37142857 -0.35714286 -0.34285714 -0.32857143 -0.31428571 -0.3 -0.28571429 -0.27142857 -0.25714286 -0.24285714 -0.22857143 -0.21428571 -0.2 -0.18571429 -0.17142857 -0.15714286 -0.14285714 -0.12857143 -0.11428571 -0.1 -0.08571429 -0.07142857 -0.05714286 -0.04285714 -0.02857143 -0.01428571 0 0 0 0 0 0
  line L9 (-25.4673, -40.7788) -> (-25.4139, -40.6879)
  arc A19 (-24.7436, -40.5025) -> (-25.4139, -40.6879) centre (-24.9829, -40.9414) ccw
  arc A20 (-24.7436, -40.5025) -> (-24.3089, -40.7306) centre (-17.3506, -26.9445) ccw
  arc A21 (-24.0808, -41.3876) -> (-24.3089, -40.7306) centre (-24.5342, -41.1769) ccw
  line L10 (-24.0808, -41.3876) -> (-24.1252, -41.4832)